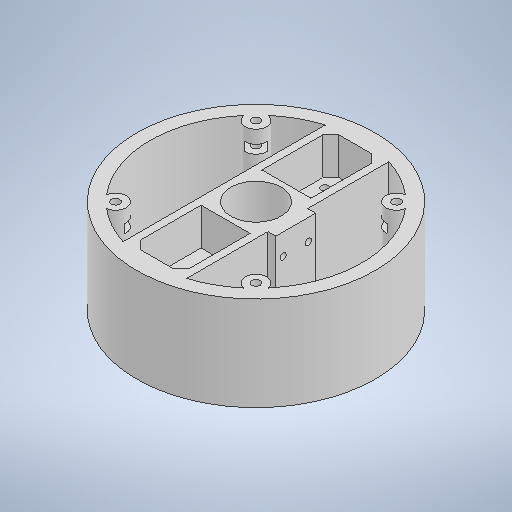
# Autodesk Inventor part: SCARA swivel top
Saved by Autodesk Inventor 2025.2 (Build 292293000, 293)
## iProperties
Created: 2025-01-26
Part Number: SCARA swivel top
Material: Generic
Document SubType Name: Modeling
Designer: caomi
Density: 1 g/cm^3
Appearance: Default
Author: caomi
Autodesk Inventor part; units mm, degrees
ref_plane "YZ Plane" through (0, 0, 0) normal (1, 0, 0) x (0, 1, 0)
ref_plane "XZ Plane" through (0, 0, 0) normal (0, 1, 0) x (-1, 0, 0)
ref_plane "XY Plane" through (0, 0, 0) normal (0, 0, 1) x (1, 0, 0)
sketch "Sketch1" plane through (0, 0, 0) normal (0, 1, 0) x (-1, 0, 0)
  circle A0 centre (0, 0) radius 45
  line L0 (9.25, 37.5) -> (-9.25, 37.5)
  line L1 (-9.25, 37.5) -> (-9.25, 11.5)
  line L2 (-9.25, 11.5) -> (9.25, 11.5)
  line L3 (9.25, 11.5) -> (9.25, 37.5)
  line L4 (-9.25, -11.5) -> (9.25, -11.5)
  line L5 (9.25, -11.5) -> (9.25, -37.5)
  line L6 (9.25, -37.5) -> (-9.25, -37.5)
  line L7 (-9.25, -37.5) -> (-9.25, -11.5)
  line L8 (22.2209, 0) -> (-22.2209, 0) construction
  circle A1 centre (0, 0) radius 3
  circle A2 centre (0, 0) radius 9.5
  line L9 (-15.5, -15.5) -> (15.5, -15.5) construction
  line L10 (15.5, -15.5) -> (15.5, 15.5) construction
  line L11 (15.5, 15.5) -> (-15.5, 15.5) construction
  line L12 (-15.5, 15.5) -> (-15.5, -15.5) construction
  line L13 (-15.5, -15.5) -> (15.5, 15.5) construction
  line L14 (15.5, -15.5) -> (-15.5, 15.5) construction
  line L15 (0, 48.862) -> (0, 10.8876) construction
  line L16 (0, -56.5383) -> (0, 11.5383) construction
  circle A3 centre (15.5, 15.5) radius 1.5
  circle A4 centre (15.5, -15.5) radius 1.5
  circle A5 centre (-15.5, -15.5) radius 1.5
  circle A6 centre (-15.5, 15.5) radius 1.5
  line L17 (-5.5, -28.5) -> (-2.9019, -30)
  line L18 (-2.9019, -30) -> (-2.9019, -33)
  line L19 (-2.9019, -33) -> (-5.5, -34.5)
  line L20 (-5.5, -34.5) -> (-8.0981, -33)
  line L21 (-8.0981, -33) -> (-8.0981, -30)
  line L22 (-8.0981, -30) -> (-5.5, -28.5)
  line L23 (5.5, -28.5) -> (8.0981, -30)
  line L24 (8.0981, -30) -> (8.0981, -33)
  line L25 (8.0981, -33) -> (5.5, -34.5)
  line L26 (5.5, -34.5) -> (2.9019, -33)
  line L27 (2.9019, -33) -> (2.9019, -30)
  line L28 (2.9019, -30) -> (5.5, -28.5)
  line L29 (-5.5, 28.5) -> (-2.9019, 30)
  line L30 (-2.9019, 30) -> (-2.9019, 33)
  line L31 (-2.9019, 33) -> (-5.5, 34.5)
  line L32 (-5.5, 34.5) -> (-8.0981, 33)
  line L33 (-8.0981, 33) -> (-8.0981, 30)
  line L34 (-8.0981, 30) -> (-5.5, 28.5)
  line L35 (5.5, 28.5) -> (8.0981, 30)
  line L36 (8.0981, 30) -> (8.0981, 33)
  line L37 (8.0981, 33) -> (5.5, 34.5)
  line L38 (5.5, 34.5) -> (2.9019, 33)
  line L39 (2.9019, 33) -> (2.9019, 30)
  line L40 (2.9019, 30) -> (5.5, 28.5)
  circle A7 centre (-5.5, -31.5) radius 1.5
  circle A8 centre (5.5, -31.5) radius 1.5
  circle A9 centre (-5.5, 31.5) radius 1.5
  circle A10 centre (5.5, 31.5) radius 1.5
  point P0 (0, 22.5)
  point P1 (0, -22.5)
  point P2 (0, -22.5)
  dimension "d0" = 90
  dimension "d11" = 6
  dimension "d12" = 19
  dimension "d13" = 31
  dimension "d14" = 26
  dimension "d15" = 18.5
  dimension "d16" = 15
  dimension "d17" = 15
  dimension "d18" = 45
  dimension "d19" = 3
  dimension "d22" = 3
  dimension "d23" = 11
  dimension "d24" = 6
  dimension "d25" = 3
  constraints: 82 end point, 18 symmetric about line, 11 centre point, 9 coincident, 6 parallel, 4 equal length, 4 equal radius, 4 horizontal, 4 midpoint, 4 vertical, 3 perpendicular, 2 point on line, 2 vertical alignment, 1 horizontal alignment, 30 other
  measures "d0" diameter of A0
  measures "d11" diameter of A1
  measures "d12" diameter of A2
  measures "d13" distance of L9.end L10.end
  measures "d14" distance of L0.end L1.end
  measures "d15" distance of L0.start L0.end
  measures "d16" distance from line of L0 point (0, 22.5)
  measures "d17" distance from line of point (0, -22.5) L6
  measures "d18" distance of point (0, -22.5) point (0, 22.5)
  measures "d19" diameter of A3
  measures "d22" distance of L20.end L21.end
  measures "d23" distance of point (-5.5, -31.5) point (5.5, -31.5)
  measures "d24" distance from line of point (-5.5, -31.5) L6
  measures "d25" diameter of A7
extrude "Extrusion1" add sketch "Sketch1" against normal blind 15 contours A0 | L3 L2 L1 L0 | L4 L5 L6 L7 | A2 | A3 | A4 | A5 | A6
extrude "Extrusion4" add sketch "Sketch1" against normal blind 3 contours L17 L18 L19 L20 L21 L22 | L23 L24 L25 L26 L27 L28 | L34 L33 L32 L31 L30 L29 | L40 L39 L38 L37 L36 L35
extrude "Extrusion2" add sketch "Sketch1" along normal blind 20.5 contours A0 | A3 | A4 | A5 | A6
extrude "Extrusion5" add sketch "Sketch1" along normal blind 6.5 contours L3 L2 L1 L0 | L4 L5 L6 L7 | L17 L18 L19 L20 L21 L22 | L23 L24 L25 L26 L27 L28 | L34 L33 L32 L31 L30 L29 | L40 L39 L38 L37 L36 L35
extrude "Extrusion3" cut sketch "Sketch1" along normal through all both and the other way through all contours A3 | A4 | A5 | A6
chamfer "Chamfer1" distance 3 angle 45 4 edges at (-9.25, 13.5, 37.5) (9.25, 13.5, 37.5) (-9.25, 13.5, -37.5) (9.25, 13.5, -37.5)
sketch "Sketch4" plane through (0, -15, 0) normal (0, -1, 0) x (1, 0, 0)
  circle A0 centre (0, 0) radius 11
  dimension "d34" = 22
  constraints: 1 centre point, 1 coincident
  measures "d34" diameter of A0
extrude "Extrusion6" cut sketch "Sketch4" against normal blind 2
sketch "Sketch5" plane through (0, 20.5, 0) normal (0, 1, 0) x (1, 0, 0)
  circle A0 centre (0, 0) radius 3 projected
  circle A1 centre (0, 0) radius 40
  line L0 (-12, -38.1576) -> (-12, 38.1576)
  line L1 (12, 38.1576) -> (12, -38.1576)
  line L2 (0, 51.8199) -> (0, 0) construction
  dimension "d37" = 80
  dimension "d38" = 12
  constraints: 6 end point, 4 point on circle, 3 vertical, 1 centre point, 1 coincident, 1 other
  measures "d37" diameter of A1
  measures "d38" distance between parallel lines of L1 L2
extrude "Extrusion7" cut sketch "Sketch5" against normal blind 30 contours A1 L1 | L0 A1
sketch "Sketch6" plane through (0, 20.5, 0) normal (0, 1, 0) x (1, 0, 0)
  circle A0 centre (-26.5165, 26.5165) radius 4
  line L0 (-26.5165, 26.5165) -> (0, 0) construction
  line L1 (-23.7305, 0) -> (26.8317, 0) construction
  circle A1 centre (-26.5165, -26.5165) radius 4
  line L2 (-26.5165, -26.5165) -> (0, 0) construction
  line L3 (0, 17.9751) -> (0, -18.8342) construction
  circle A2 centre (26.5165, 26.5165) radius 4
  circle A3 centre (26.5165, -26.5165) radius 4
  line L4 (-23.0589, 27.443) -> (-23.9854, 23.9854)
  line L5 (-23.9854, 23.9854) -> (-27.443, 23.0589)
  line L6 (-27.443, 23.0589) -> (-29.9741, 25.59)
  line L7 (-29.9741, 25.59) -> (-29.0476, 29.0476)
  line L8 (-29.0476, 29.0476) -> (-25.59, 29.9741)
  line L9 (-25.59, 29.9741) -> (-23.0589, 27.443)
  circle A4 centre (-26.5165, 26.5165) radius 1.6
  line L10 (0, -17.9751) -> (0, 18.8342) construction
  line L11 (-23.0589, -27.443) -> (-23.9854, -23.9854)
  line L12 (-23.9854, -23.9854) -> (-27.443, -23.0589)
  line L13 (-27.443, -23.0589) -> (-29.9741, -25.59)
  line L14 (-29.9741, -25.59) -> (-29.0476, -29.0476)
  line L15 (-29.0476, -29.0476) -> (-25.59, -29.9741)
  line L16 (-25.59, -29.9741) -> (-23.0589, -27.443)
  circle A5 centre (-26.5165, -26.5165) radius 1.6
  line L17 (23.0589, 27.443) -> (23.9854, 23.9854)
  line L18 (23.9854, 23.9854) -> (27.443, 23.0589)
  line L19 (27.443, 23.0589) -> (29.9741, 25.59)
  line L20 (29.9741, 25.59) -> (29.0476, 29.0476)
  line L21 (29.0476, 29.0476) -> (25.59, 29.9741)
  line L22 (25.59, 29.9741) -> (23.0589, 27.443)
  circle A6 centre (26.5165, 26.5165) radius 1.6
  line L23 (29.9741, -25.59) -> (29.0476, -29.0476)
  line L24 (27.443, -23.0589) -> (29.9741, -25.59)
  line L25 (23.9854, -23.9854) -> (27.443, -23.0589)
  circle A7 centre (26.5165, -26.5165) radius 1.6
  line L26 (23.0589, -27.443) -> (23.9854, -23.9854)
  line L27 (25.59, -29.9741) -> (23.0589, -27.443)
  line L28 (29.0476, -29.0476) -> (25.59, -29.9741)
  line L29 (-27.443, 23.0589) -> (-26.9211, 22.537)
  line L30 (-23.0589, 27.443) -> (-22.537, 26.9211)
  line L31 (-27.443, -23.0589) -> (-26.9211, -22.537)
  line L32 (-23.0589, -27.443) -> (-22.537, -26.9211)
  line L33 (27.443, 23.0589) -> (26.9211, 22.537)
  line L34 (23.0589, 27.443) -> (22.537, 26.9211)
  line L35 (27.443, -23.0589) -> (26.9211, -22.537)
  line L36 (23.0589, -27.443) -> (22.537, -26.9211)
  point P0 (22.537, 26.9211)
  point P1 (26.9211, 22.537)
  point P2 (26.9211, -22.537)
  point P3 (22.537, -26.9211)
  point P4 (-22.537, -26.9211)
  dimension "d41" = 37.5
  dimension "d43" = 8
  dimension "d44" = 45
  dimension "d45" = 6.2
  dimension "d46" = 3.2
  constraints: 74 end point, 31 symmetric about line, 8 centre point, 2 coincident, 2 collinear, 2 point on circle, 2 point on line, 1 equal radius, 1 horizontal, 1 vertical, 20 other
  measures "d41" distance of L0.start L0.end
  measures "d43" diameter of A0
  measures "d44" angle of L1 L0
  measures "d45" distance between parallel lines of L8 L5
  measures "d46" diameter of A4
extrude "Extrusion8" add sketch "Sketch6" against normal up to surface (30 mm away)
ref_plane "Work Plane1" through (0, 15.5, 0) normal (0, 1, 0) x (1, 0, 0)
extrude "Extrusion9" cut sketch "Sketch6" against normal blind 3.2 from surface at -5 contours A0 L29 L5 L4 L30 | L4 L5 L6 L7 L8 L9 | A1 L32 L11 L12 L31 | L12 L11 L16 L15 L14 L13 | L34 L17 L18 L33 A2 | L22 L21 L20 L19 L18 L17 | L35 L25 L26 L36 A3 | L24 L23 L28 L27 L26 L25
sketch "Sketch7" plane through (0, -9.5, 0) normal (0, 1, 0) x (1, 0, 0)
  line L0 (-18.5591, 0) -> (20.3221, 0) construction
  line L1 (12, -38.1576) -> (12, 38.1576) projected
  line L2 (12, 7.5) -> (15, 7.5)
  line L3 (15, 7.5) -> (15, -7.5)
  line L4 (15, -7.5) -> (12, -7.5)
  line L5 (12, -7.5) -> (12, 7.5)
  point P0 (0, 0)
  dimension "d61" = 15
  dimension "d62" = 3
  constraints: 10 end point, 2 horizontal, 2 parallel, 2 point on line, 1 perpendicular, 1 other
  measures "d61" distance of L2.end L3.end
  measures "d62" distance between parallel lines of L1 L3
extrude "Extrusion10" add sketch "Sketch7" along normal up to surface (30 mm away)
sketch "Sketch8" plane through (15, -9.5, -7.5) normal (-1, 0, 0) x (0, 0, 1)
  circle A0 centre (12.25, 22) radius 1.2
  circle A1 centre (2.75, 22) radius 1.2
  line L0 (2.75, 22) -> (12.25, 22) construction
  line L1 (7.5, 28.9581) -> (7.5, 20.5932) construction
  line L2 (0, 30) -> (15, 30) projected
  point P0 (7.5, 9.5)
  point P1 (7.5, 30)
  dimension "d56" = 9.5
  dimension "d57" = 2.4
  dimension "d63" = 8
  constraints: 4 end point, 2 centre point, 1 equal radius, 1 horizontal, 1 point on line, 1 vertical, 1 other
  measures "d56" distance of L0.start L0.end
  measures "d57" diameter of A1
  measures "d63" distance between parallel lines of L0 L2
extrude "Extrusion11" cut sketch "Sketch8" along normal blind 5
equation "\"d17\" = d16"
body "Solid1"
